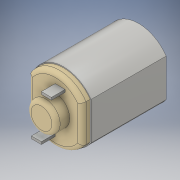
# Autodesk Inventor part: J024 motor
Saved by Autodesk Inventor 2016 SP1 (Build 200210100, 210)
## iProperties
Created: 2016-09-17
Part Number: J024 motor
Material: Generic
Document SubType Name: Modeling
Designer: benja
Density: 1 g/cm^3
Appearance: Default
Author: benja
Autodesk Inventor part; units mm, degrees
ref_plane "YZ Plane" through (0, 0, 0) normal (1, 0, 0) x (0, 1, 0)
ref_plane "XZ Plane" through (0, 0, 0) normal (0, 1, 0) x (-1, 0, 0)
ref_plane "XY Plane" through (0, 0, 0) normal (0, 0, 1) x (1, 0, 0)
sketch "Sketch1" plane through (0, 0, 0) normal (0, 0, 1) x (1, 0, 0)
  point P0 (0, 0)
sketch "Sketch2" plane through (0, 0, 0) normal (0, 0, 1) x (1, 0, 0)
  line L0 (-3.3, 2.2605) -> (-3.3, -2.2605)
  line L1 (3.3, 2.2605) -> (3.3, -2.2605)
  arc A0 (-3.3, -2.2605) -> (3.3, -2.2605) centre (0, 0) ccw
  arc A1 (3.3, 2.2605) -> (-3.3, 2.2605) centre (0, 0) ccw
  dimension "d1" = 6.6
  dimension "d2" = 4
  constraints: 4 end point, 4 point on circle, 2 centre point, 2 parallel, 1 coincident, 1 concentric, 1 vertical
  measures "d1" distance between parallel lines of L1 L0
  measures "d2" radius of A1
extrude "Extrusion1" add sketch "Sketch2" along normal blind 9
sketch "Sketch3" plane through (0, 0, 9) normal (0, 0, 1) x (1, 0, 0)
  point P0 (0, 0)
sketch "Sketch4" plane through (0, 0, 9) normal (0, 0, 1) x (1, 0, 0)
  line L0 (-3.3, 2.2605) -> (-3.3, -2.2605) projected
  arc A0 (-3.3, -2.2605) -> (3.3, -2.2605) centre (0, 0) ccw projected
  line L1 (3.3, -2.2605) -> (3.3, 2.2605) projected
  arc A1 (3.3, 2.2605) -> (-3.3, 2.2605) centre (0, 0) ccw projected
  line L2 (-3.2, 2.2293) -> (-3.2, -2.2293)
  arc A2 (-3.2, -2.2293) -> (3.2, -2.2293) centre (0, 0) ccw
  line L3 (3.2, -2.2293) -> (3.2, 2.2293)
  arc A3 (3.2, 2.2293) -> (-3.2, 2.2293) centre (0, 0) ccw
  dimension "d5" = 0.1
  constraints: 4 end point, 4 point on circle, 2 centre point, 3 other
  measures "d5" radial gap between concentric circles of A1 A3
extrude "Extrusion2" add sketch "Sketch4" along normal blind 1 contours A3 L3 A2 L2
fillet "Fillet1" radius 0.5 4 edges at (3.2, 0, 10) (0, 3.9, 10) (-3.2, 0, 10) (0, -3.9, 10)
sketch "Sketch5" plane through (0, 0, 10) normal (0, 0, 1) x (1, 0, 0)
  circle A0 centre (0, 0) radius 1.75
  dimension "d9" = 3.5
  constraints: 1 centre point, 1 coincident
  measures "d9" diameter of A0
extrude "Extrusion3" add sketch "Sketch5" along normal blind 1.65
fillet "Fillet2" radius 0.5 1 edges at (-1.75, 0, 11.65)
sketch "Sketch6" plane through (0, 0, 10) normal (0, 0, 1) x (1, 0, 0)
  circle A0 centre (0, 0) radius 1.75 projected
  line L0 (0, -2.75) -> (-1.2, -2.75)
  line L1 (-1.2, -2.75) -> (-1.2, -2.45)
  line L2 (-1.2, -2.45) -> (0, -2.45)
  line L3 (0, -2.45) -> (0, -2.75)
  line L4 (0, 2.45) -> (1.2, 2.45)
  line L5 (1.2, 2.45) -> (1.2, 2.75)
  line L6 (1.2, 2.75) -> (0, 2.75)
  line L7 (0, 2.75) -> (0, 2.45)
  point P0 (1.4682, 1.2)
  dimension "d21" = 1.2
  dimension "d22" = 0.3
  dimension "d23" = 1.2
  dimension "d24" = 0.3
  dimension "d25" = 0.7
  dimension "d26" = 0.7
  constraints: 16 end point, 4 parallel, 2 horizontal, 2 perpendicular, 2 point on line
  measures "d21" distance of L1.end L2.end
  measures "d22" distance of L0.end L1.end
  measures "d23" distance of L4.start L4.end
  measures "d24" distance of L4.end L5.end
  measures "d25" distance edge to line of A0 L4
  measures "d26" distance edge to line of A0 L2
extrude "Extrusion4" add sketch "Sketch6" along normal blind 1.65 contours L0 L1 L2 L3 | L7 L6 L5 L4
body "Solid1"
